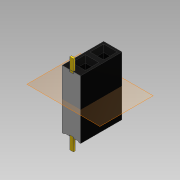
# Autodesk Inventor part: SSM-101-F-DH
Saved by Autodesk Inventor 2016 (Build 200138000, 138)
## iProperties
Created: 2016-05-29
Part Number: SSM-101-F-DH
Material: Generic
Document SubType Name: Modeling
Designer: admin
Density: 1 g/cm^3
Appearance: Default
Mass: 0.10342 g
Surface Area: 2.21165 cm^2
Volume: 0.10342 cm^3
Author: admin
Autodesk Inventor part; units mm, degrees
ref_plane "YZ Plane" through (0, 0, 0) normal (1, 0, 0) x (0, 1, 0)
ref_plane "XZ Plane" through (0, 0, 0) normal (0, 1, 0) x (-1, 0, 0)
sketch "Sketch1" plane through (0, 0, 0) normal (0, 1, 0) x (-1, 0, 0)
  line L0 (-1.27, -4.065) -> (-1.27, 4.065)
  line L1 (-1.27, 4.065) -> (1.27, 4.065)
  line L2 (1.27, 4.065) -> (1.27, -4.065)
  line L3 (1.0272, -4.065) -> (0.8972, -3.935)
  line L4 (0.8972, -3.935) -> (-0.8972, -3.935)
  line L5 (-0.8972, -3.935) -> (-1.0272, -4.065)
  line L6 (1.27, -4.065) -> (1.0272, -4.065)
  line L7 (-1.0272, -4.065) -> (-1.27, -4.065)
  line L8 (0, -2.6831) -> (0, -0.9898) construction
  point P0 (0, 0)
  point P1 (0, 4.065)
  point P2 (1.27, 0)
  point P3 (0, -3.935)
  dimension "d1" = 2.54
  dimension "d2" = 0.13
  dimension "d3" = 8.13
  dimension "d4" = 45
  constraints: 18 end point, 3 horizontal, 3 midpoint, 3 parallel, 2 perpendicular, 2 vertical alignment, 1 collinear, 1 horizontal alignment, 1 point on line, 1 vertical, 1 other
  measures "d1" distance between parallel lines of L0 L2
  measures "d2" distance between parallel lines of L4 L6
  measures "d3" distance between parallel lines of L1 L6
  measures "d4" angle of L4 L3
extrude "Extrusion1" add sketch "Sketch1" along normal blind 5.08
sketch "Sketch2" plane through (-1.27, 0, 4.065) normal (0, 0, 1) x (1, 0, 0)
  line L0 (0.825, 4.255) -> (1.715, 4.255)
  line L1 (1.715, 4.255) -> (1.715, 3.365)
  line L2 (1.715, 3.365) -> (0.825, 3.365)
  line L3 (0.825, 3.365) -> (0.825, 4.255)
  line L4 (0.825, 1.715) -> (1.715, 1.715)
  line L5 (1.715, 1.715) -> (1.715, 0.825)
  line L6 (1.715, 0.825) -> (0.825, 0.825)
  line L7 (0.825, 0.825) -> (0.825, 1.715)
  line L8 (0.4511, 3.81) -> (2.2201, 3.81) construction
  line L9 (2.2201, 1.27) -> (0.4335, 1.27) construction
  line L10 (0, 0) -> (2.54, 0) projected
  line L11 (2.54, 0) -> (2.54, 5.08) projected
  line L12 (0, 5.08) -> (2.54, 5.08) projected
  line L13 (0, 0) -> (0, 5.08) projected
  point P0 (1.27, 0)
  point P1 (0.825, 3.81)
  point P2 (0.825, 1.27)
  point P3 (1.27, 5.08)
  point P4 (1.27, 4.255)
  point P5 (1.27, 1.715)
  dimension "d7" = 2.54
  dimension "d8" = 0.89
  dimension "d9" = 1.27
  constraints: 20 end point, 5 midpoint, 4 horizontal, 4 parallel, 3 equal length, 3 point on line, 2 perpendicular, 2 vertical alignment
  measures "d7" distance between parallel lines of L9 L8
  measures "d8" distance of L1.end L2.end
  measures "d9" distance between parallel lines of L12 L8
extrude "Extrusion2" cut sketch "Sketch2" against normal blind 8 contours L0 L1 L2 L3 | L4 L5 L6 L7
sketch "Sketch3" plane through (0, 0, 0) normal (1, 0, 0) x (0, 1, 0)
  line L0 (0, 4.065) -> (5.08, 4.065) projected
  line L1 (5.08, -4.065) -> (5.08, 4.065) projected
  line L2 (0, -3.935) -> (5.08, -3.935) projected
  line L3 (-0.39, 5.59) -> (-0.64, 5.59)
  line L4 (-0.64, 5.59) -> (-0.64, 3.7923)
  line L5 (-0.64, 3.7923) -> (-0.2868, 3.7923)
  line L6 (-0.39, 4.0423) -> (-0.39, 5.59)
  line L7 (-0.39, -3.7923) -> (-0.64, -3.7923)
  line L8 (-0.64, -3.7923) -> (-0.64, -5.59)
  line L9 (-0.64, -5.59) -> (-0.39, -5.59)
  line L10 (-0.39, -5.59) -> (-0.39, -4.0423)
  line L11 (-1.3876, 0) -> (-0.3881, 0) construction
  line L12 (0, -4.065) -> (0, 4.065) projected
  line L13 (-0.39, -3.7923) -> (0, -3.7923)
  line L14 (0, -3.7923) -> (0, -4.0423)
  line L15 (0, -4.0423) -> (-0.39, -4.0423)
  line L16 (-0.39, 4.0423) -> (0, 4.0423)
  line L17 (0, 4.0423) -> (0, 3.7923)
  line L18 (0, 3.7923) -> (-0.2868, 3.7923)
  point P0 (0, 0)
  dimension "d30" = 0.25
  dimension "d31" = 11.18
  dimension "d34" = 5.72
  constraints: 30 end point, 7 horizontal, 4 collinear, 4 parallel, 3 equal length, 2 perpendicular, 2 vertical, 1 point on line, 1 other
  measures "d30" distance of L3.start L3.end
  measures "d31" distance between parallel lines of L9 L3
  measures "d34" distance between parallel lines of L8 L1
ref_plane "Work Plane1" through (-1.27, 0, 3.94) normal (0, 0, 1) x (1, 0, 0)
extrude "Extrusion3" add sketch "Sketch3" along normal mid plane 0.51 contours L12 L18 L5 L4 L3 L6 L16 | L12 L15 L10 L9 L8 L7 L13
chamfer "Chamfer1" distance 0.5 angle 45 8 edges at (0.445, 3.81, 4.065) (0, 3.365, 4.065) (-0.445, 3.81, 4.065) (0, 4.255, 4.065) (0, 1.715, 4.065) (0.445, 1.27, 4.065) (0, 0.825, 4.065) (-0.445, 1.27, 4.065)
ref_plane "Work Plane3" through (-0.255, -0.64, 0) normal (0, 0, 1) x (1, 0, 0)
sketch "Sketch6" plane through (0, 0, 0) normal (0, -1, 0) x (1, 0, 0)
  line L0 (0.255, -3.7923) -> (0.255, -3.935) projected
  line L1 (0.8972, -3.935) -> (0.255, -3.935) projected
  line L2 (1.0272, -4.065) -> (0.8972, -3.935) projected
  line L3 (1.27, -4.065) -> (1.0272, -4.065) projected
  line L4 (1.27, 4.065) -> (1.27, -4.065) projected
  line L5 (-1.27, 4.065) -> (1.27, 4.065) projected
  line L6 (-1.27, -4.065) -> (-1.27, 4.065) projected
  line L7 (-1.0272, -4.065) -> (-1.27, -4.065) projected
  line L8 (-0.8972, -3.935) -> (-1.0272, -4.065) projected
  line L9 (-0.255, -3.935) -> (-0.8972, -3.935) projected
  line L10 (-0.255, -3.935) -> (-0.255, -3.7923) projected
  line L11 (-0.255, -3.7923) -> (0.255, -3.7923) projected
  line L12 (-0.255, 3.7923) -> (-0.255, 4.0423) projected
  line L13 (-0.255, 4.0423) -> (0.255, 4.0423) projected
  line L14 (0.255, 4.0423) -> (0.255, 3.7923) projected
  line L15 (0.255, 3.7923) -> (-0.255, 3.7923) projected
  point P0 (0, 0)
extrude "Extrusion4" add sketch "Sketch6" along normal blind 0.65
body "Solid1"
